Autodesk Fusion 360 part; units mm, degrees
(part 2 of 2)
  spline S324 degree 3 poles (60.198324, 30.761501) (59.837342, 30.709202) (59.46806, 30.741093) (59.101979, 30.761501) knots 0 0 0 0 1 1 1 1
  line L63 (59.101979, 30.761501) -> (58.561134, 30.761501)
  spline S325 degree 3 poles (58.561134, 30.761501) (58.184845, 30.716219) (57.990316, 30.52169) (57.963534, 29.991064) knots 0 0 0 0 1 1 1 1
  spline S326 degree 3 poles (57.963534, 29.991064) (57.908685, 28.917676) (57.673984, 27.860871) (57.363384, 26.828299) knots 0 0 0 0 1 1 1 1
  spline S327 degree 3 poles (57.363384, 26.828299) (56.554039, 24.131112) (55.522741, 21.519391) (54.262484, 18.999518) knots 0 0 0 0 1 1 1 1
  spline S328 degree 3 poles (54.262484, 18.999518) (54.040531, 18.554979) (53.851111, 18.106625) (54.579458, 18.083658) knots 0 0 0 0 1 1 1 1
  spline S329 degree 3 poles (54.579458, 18.083658) (55.94368, 18.041568) (57.30981, 18.077284) (58.675298, 18.084301) knots 0 0 0 0 1 1 1 1
  spline S330 degree 3 poles (58.675298, 18.084301) (61.78194, 18.102159) (64.888582, 18.151908) (67.993939, 18.127666) knots 0 0 0 0 1 1 1 1
  spline S331 degree 3 poles (67.993939, 18.127666) (69.479351, 18.116172) (69.55014, 18.163372) (68.902791, 19.494428) knots 0 0 0 0 1 1 1 1
  line L64 (56.440518, 31.1244) -> (56.652262, 31.1244)
  line L65 (56.652262, 31.1244) -> (57.340426, 31.1244)
  line L66 (57.340426, 31.1244) -> (60.593756, 31.1244)
  line L67 (60.593756, 31.1244) -> (65.011037, 31.1244)
  line L68 (65.011037, 31.1244) -> (66.259811, 31.1244)
  line L69 (66.259811, 31.1244) -> (66.87017, 31.1244)
  line L70 (66.87017, 31.1244) -> (66.978592, 31.1244)
  spline S332 degree 3 poles (66.978592, 31.1244) (66.9939, 31.126317) (67.007291, 31.130141) (67.021956, 31.132049) knots 0 0 0 0 1 1 1 1
  spline S333 degree 3 poles (67.021956, 31.132049) (67.869567, 31.209222) (68.532866, 31.920344) (68.532866, 32.788371) knots 0 0 0 0 1 1 1 1
  spline S334 degree 3 poles (68.532866, 32.788371) (68.532866, 33.70678) (67.788569, 34.45171) (66.87017, 34.45171) knots 0 0 0 0 1 1 1 1
  line L71 (66.87017, 34.45171) -> (65.867571, 34.45171)
  spline S335 degree 3 poles (65.867571, 34.45171) (65.840147, 34.522499) (65.821647, 34.611798) (65.813355, 34.725319) knots 0 0 0 0 1 1 1 1
  spline S336 degree 3 poles (65.813355, 34.725319) (65.738732, 35.740034) (66.023182, 36.760481) (65.736824, 37.770096) knots 0 0 0 0 1 1 1 1
  line L72 (65.736824, 37.770096) -> (57.742213, 37.770096)
  spline S337 degree 3 poles (57.742213, 37.770096) (57.471154, 37.589601) (57.487104, 37.30515) (57.489011, 37.028991) knots 0 0 0 0 1 1 1 1
  spline S338 degree 3 poles (57.489011, 37.028991) (57.492203, 36.493256) (57.49922, 35.956878) (57.49922, 35.421143) knots 0 0 0 0 1 1 1 1
  spline S339 degree 3 poles (57.49922, 35.421143) (57.498578, 35.044211) (57.500495, 34.697263) (57.326383, 34.451077) knots 0 0 0 0 1 1 1 1
  line L73 (57.326383, 34.451077) -> (56.441783, 34.451077)
  spline S340 degree 3 poles (56.441783, 34.451077) (55.522099, 34.451077) (54.777811, 33.70678) (54.777811, 32.787739) knots 0 0 0 0 1 1 1 1
  spline S341 degree 3 poles (54.777811, 32.787739) (54.777811, 31.868697) (55.520192, 31.1244) (56.440518, 31.1244) knots 0 0 0 0 1 1 1 1
  line L74 (-8.552116, 16.552331) -> (9.004772, 16.552331)
  line L75 (0.226328, 16.552331) -> (0.226328, 70.000001)
  line L76 (0.226328, 16.552331) -> (0, 0)
  spline S342 degree 5 poles (3.604041, 35.067921) (3.593764, 35.084393) (3.57371, 35.118054) (3.545124, 35.170701) (3.510208, 35.245502) (3.474499, 35.350437) (3.456283, 35.449296) (3.451368, 35.536039) (3.452601, 35.600364) (3.454346, 35.634152) knots 0 0 0 0 0 0 0.2 0.4 0.6 0.8 1 1 1 1 1 1
  spline S343 degree 5 poles (9.004772, 16.552331) (9.002751, 16.530164) (9.001516, 16.48807) (9.008084, 16.431645) (9.031355, 16.36799) (9.076547, 16.301267) (9.120604, 16.254192) (9.156631, 16.221268) (9.18189, 16.200308) (9.194829, 16.190075) knots 0 0 0 0 0 0 0.2 0.4 0.6 0.8 1 1 1 1 1 1
  spline S344 degree 5 poles (9.543699, 13.760124) (9.538967, 13.770504) (9.530393, 13.791743) (9.520207, 13.825034) (9.512346, 13.872487) (9.516718, 13.939409) (9.538733, 14.002866) (9.570891, 14.058841) (9.600397, 14.100479) (9.617169, 14.12238) knots 0 0 0 0 0 0 0.2 0.4 0.6 0.8 1 1 1 1 1 1
  spline S345 degree 5 poles (10.207632, 3.20609) (10.210363, 3.188817) (10.218178, 3.155107) (10.236952, 3.107041) (10.274139, 3.047265) (10.334108, 2.977329) (10.388702, 2.923726) (10.432148, 2.884411) (10.46215, 2.858569) (10.477412, 2.845741) knots 0 0 0 0 0 0 0.2 0.4 0.6 0.8 1 1 1 1 1 1
  line L77 (10.201047, 3.247726) -> (10.214216, 3.164454)
  line L78 (9.576458, 14.06922) -> (9.657879, 14.175541)
  line L79 (9.009544, 16.604663) -> (9, 16.5)
  line L80 (3.45, 35.549999) -> (3.458692, 35.718305)
  spline S346 degree 5 poles (0.925268, 60.472399) (0.927849, 60.442545) (0.934441, 60.38556) (0.948615, 60.308246) (0.97532, 60.21933) (1.020307, 60.124567) (1.066325, 60.057773) (1.107871, 60.011814) (1.139078, 59.983026) (1.15556, 59.969095) knots 0 0 0 0 0 0 0.2 0.4 0.6 0.8 1 1 1 1 1 1
  line L81 (0.918097, 60.555341) -> (0.932438, 60.389457)
  line L82 (1.110579, 60.007114) -> (1.200541, 59.931076)
  line L83 (-0.702904, 59.969095) -> (-0.725484, 59.95001)
  spline S347 degree 5 poles (-0.477532, 60.425537) (-0.479901, 60.406523) (-0.486572, 60.36092) (-0.500338, 60.293952) (-0.525574, 60.2132) (-0.567651, 60.124567) (-0.613668, 60.057773) (-0.655214, 60.011814) (-0.686422, 59.983026) (-0.702904, 59.969095) knots 0.06468932 0.06468932 0.06468932 0.06468932 0.06468932 0.06468932 0.2 0.4 0.6 0.8 1 1 1 1 1 1
  line L84 (-0.46874, 60.496097) -> (-0.486323, 60.354978)
  line L85 (-0.662071, 60.003607) -> (-0.743736, 59.934583)
  spline S348 degree 5 poles (4.037624, 32.930053) (4.022709, 32.601004) (4.008606, 31.970034) (4.034587, 31.104885) (4.150496, 30.091536) (4.385544, 28.980369) (4.617829, 28.167758) (4.808756, 27.587129) (4.942985, 27.212022) (5.011837, 27.027466) knots 0 0 0 0 0 0 0.2 0.4 0.6 0.8 1 1 1 1 1 1
  line L86 (4.075249, 33.760107) -> (4, 32.099999)
  constraint perpendicular L74 L75
  constraint coincident L76.end origin
revolve "Revolve1" add sketch "King" angle 360 about axis through (0, 0.226328, 16.552331) along (0, 0, 1) contours S296 S297 S298 S299 S300 L58 L59 S312 S313 S314 S315 S316 L60 S317 S318 S319 S320 L75 | S113 L9 L58 L75 S342 | L8 S111 S112 S113 L9 L74 L75 L79 S348 | S112 S348 picked at (1.75805, 46.98267) picked at (2.208838, 35.513189) picked at (1.592253, 27.050987) picked at (4.172625, 31.277112) makes body 1
revolve "Revolve2" add sketch "King" angle 360 about axis through (0, 0.226328, 16.552331) along (0, -0.01367222, -0.99990653) contours L8 L11 L74 L76 S343 | L10 S119 S120 S121 L11 L76 | L10 L13 L76 S344 | L12 S125 S126 S127 L13 L76 | L12 L15 L76 S345 | L15 S135 S136 S137 S138 L76 picked at (3.150369, 16.412485) picked at (6.335033, 14.811612) picked at (3.299017, 13.923055) picked at (3.674609, 9.616021) picked at (3.430127, 3.085973) picked at (3.476174, 1.183926) bodies 1
extrude "Extrude1" add sketch "King" along normal mid plane 6.4 separate body contours S27 S28 S29 S30 S31 S32 S43 S44 S45 S46 S47 S48 S49 S50 L75 | S32 S33 S34 S35 S36 S37 S38 S39 S40 S41 S42 S43 L75 picked at (-2.855966, 64.723087) picked at (3.071571, 64.690888) makes body 2
extrude "Extrude2" add sketch "King" along normal mid plane 3.2 contours S43 S300 L75 L83 S347 L85 | S43 S300 L75 S346 picked at (-0.145181, 60.183621) picked at (0.596915, 60.184877) bodies 1 2
extrude "Extrude3" cut sketch "King" along normal mid plane 20 contours S112 S348 picked at (4.172625, 31.277112) bodies 1
pattern_circular "C-Pattern1" count 6 over 360 about axis through (0, 0.226328, 16.552331) along (0, 0, 1) of "Extrude3"
named bodies: "King"
